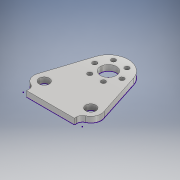
# Autodesk Inventor part: LR3
Saved by Autodesk Inventor 2018 (Build 220112000, 112)
## iProperties
Created: 2020-04-08
Part Number: LR3
Material: Типовые
Document SubType Name: Modeling
Designer: Siarhei
Density: 1 g/cm^3
Appearance: По умолчанию
Author: Siarhei
Autodesk Inventor part; units mm, degrees
ref_plane "YZ Plane" through (0, 0, 0) normal (1, 0, 0) x (0, 1, 0)
ref_plane "XZ Plane" through (0, 0, 0) normal (0, 1, 0) x (-1, 0, 0)
ref_plane "XY Plane" through (0, 0, 0) normal (0, 0, 1) x (1, 0, 0)
sketch "Эскиз1" plane through (0, 0, 0) normal (0, 0, 1) x (1, 0, 0)
  line L0 (0, 0) -> (84, 0)
  circle A0 centre (1, 30) radius 9
  circle A1 centre (83, 30) radius 9
  circle A2 centre (42, 102) radius 14
  circle A3 centre (18, 102) radius 4
  circle A4 centre (66, 102) radius 4
  circle A5 centre (30, 122.7846) radius 4
  circle A6 centre (54, 81.2154) radius 4
  circle A7 centre (54, 122.7846) radius 4
  circle A8 centre (30, 81.2154) radius 4
  arc A9 (90.0714, 13.4472) -> (83, 48) centre (83, 30) ccw
  arc A10 (1, 48) -> (-6.0714, 13.4472) centre (1, 30) ccw
  line L1 (84, 0) -> (84, 4.2512)
  line L2 (0, 0) -> (0, 4.2512)
  arc A11 (0, 4.2512) -> (-6.0714, 13.4472) centre (-10, 4.2512) ccw
  arc A12 (90.0714, 13.4472) -> (84, 4.2512) centre (94, 4.2512) ccw
  line L3 (83, 48) -> (64, 48)
  line L4 (56, 63.9343) -> (56, 56)
  line L5 (1, 48) -> (20, 48)
  line L6 (28, 63.9343) -> (28, 56)
  arc A13 (20, 48) -> (28, 56) centre (20, 56) ccw
  arc A14 (56, 56) -> (64, 48) centre (64, 56) ccw
  arc A15 (60.6667, 72.3933) -> (56, 63.9343) centre (66, 63.9343) ccw
  arc A16 (28, 63.9343) -> (23.3333, 72.3933) centre (18, 63.9343) ccw
  circle A17 centre (42, 102) radius 35
  line L7 (74.8961, 113.9519) -> (99.7811, 36.5112)
  line L8 (8.6749, 112.6974) -> (-15.7811, 36.5112)
  point P0 (84, 12.0278)
  point P1 (0, 12.0278)
  point P2 (56, 69.922)
  point P3 (28, 69.922)
  dimension "d0" = 84
  dimension "d2" = 18
  dimension "d3" = 18
  dimension "d4" = 82
  dimension "d5" = 28
  dimension "d6" = 8
  dimension "d7" = 8
  dimension "d8" = 8
  dimension "d9" = 8
  dimension "d10" = 8
  dimension "d11" = 8
  dimension "d12" = 18
  dimension "d13" = 10
  dimension "d14" = 10
  dimension "d16" = 8
  dimension "d17" = 8
  dimension "d18" = 10
  dimension "d19" = 10
  dimension "d20" = 70
  dimension "d21" = 30
  dimension "d22" = 72
  dimension "d23" = 28
  dimension "d134" = 17.814
  dimension "d135" = 35.611
  dimension "d136" = 28
  dimension "d137" = 106.1669
  dimension "d138" = 15.7811
  dimension "d139" = 12.126
  dimension "d140" = 18
  dimension "d141" = 26.2614
  dimension "d142" = 31.4603
  dimension "d143" = 17.1919
  dimension "d144" = 30
  dimension "d145" = 29.9094
  dimension "d146" = 30
  dimension "d147" = 40.0412
  dimension "d148" = 54
  dimension "d149" = 52.7587
  dimension "d150" = 54
  dimension "d151" = 58.1178
  dimension "d152" = 61.8047
  dimension "d153" = 57.8246
  dimension "d154" = 66
  dimension "d155" = 90.5299
  dimension "d156" = 90.5299
  constraints: 22 point on circle, 18 centre point, 18 end point, 17 tangent, 4 point on line, 3 coincident, 3 horizontal, 2 perpendicular, 1 concentric, 1 equal radius, 1 parallel, 1 vertical
  measures "d0" distance of L0.start L0.end
  measures "d2" diameter of A0
  measures "d3" diameter of A1
  measures "d4" distance of A1.centre A0.centre
  measures "d5" diameter of A2
  measures "d6" diameter of A3
  measures "d7" diameter of A4
  measures "d8" diameter of A5
  measures "d9" diameter of A6
  measures "d10" diameter of A7
  measures "d11" diameter of A8
  measures "d12" radius of A9
  measures "d13" radius of A11
  measures "d14" radius of A12
  measures "d16" radius of A13
  measures "d17" radius of A14
  measures "d18" radius of A15
  measures "d19" radius of A16
  measures "d20" diameter of A17
  measures "d21" vertical distance of L0.end A1.centre
  measures "d22" vertical distance of A2.centre A1.centre
  measures "d23" distance of L4.end L6.end
  measures "d134" angle of L7 L1
  measures "d135" angle of L7 L8
  measures "d136" distance between parallel lines of L1 L4
  measures "d137" distance from line of L0.start L7
  measures "d138" distance from line of L7.end L1
  measures "d139" distance from line of A4.centre L7
  measures "d140" distance from line of A4.centre L1
  measures "d141" distance from line of A15.start L7
  measures "d142" distance from line of point (56, 69.922) L7
  measures "d143" distance from line of A7.centre L7
  measures "d144" distance from line of A7.centre L1
  measures "d145" distance from line of A6.centre L7
  measures "d146" distance from line of A6.centre L1
  measures "d147" distance from line of A5.centre L7
  measures "d148" distance from line of A5.centre L1
  measures "d149" distance from line of A8.centre L7
  measures "d150" distance from line of A8.centre L1
  measures "d151" distance from line of point (28, 69.922) L7
  measures "d152" distance from line of A16.end L7
  measures "d153" distance from line of A3.centre L7
  measures "d154" distance from line of A3.centre L1
  measures "d155" distance from line of A10.start L7
  measures "d156" distance from line of L5.start L7
extrude "Выдавливание1" add sketch "Эскиз1" along normal blind 10 contours L2 A11 A10 L5 A13 L6 A16 A17 A15 L4 A14 L3 A9 A12 L1 L0 | L8 A17 A16 L6 A13 L5 A10 | A9 L3 A14 L4 A15 A17 L7 | A17 L7 picked at (19.1339, 115.3288)
